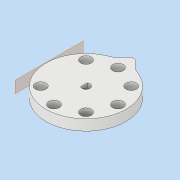
# Autodesk Inventor part: servo horn
Saved by Autodesk Inventor 2017 SP1 (Build 210196100, 196)
## iProperties
Created: 2018-12-30
Part Number: servo horn
Material: Generic
Document SubType Name: Modeling
Designer: Dylan Rice
Density: 1 g/cm^3
Appearance: Default
Author: Dylan Rice
Autodesk Inventor part; units mm, degrees
ref_plane "XZ Plane" through (0, 0, 0) normal (0, 1, 0) x (-1, 0, 0)
ref_plane "XY Plane" through (0, 0, 0) normal (0, 0, 1) x (1, 0, 0)
sketch "Sketch1" plane through (0, 0, 0) normal (0, 1, 0) x (-1, 0, 0)
  arc A0 (0.8292, 1.25) -> (0.8292, -1.25) centre (0, 0) ccw
  line L0 (0.8292, 1.25) -> (0.8292, -1.25)
  circle A1 centre (0, 0) radius 15 construction
  circle A2 centre (0, 0) radius 18 construction
  line L1 (0, -15) -> (0, -18) construction
  arc A3 (-1, -17.618) -> (1, -17.618) centre (0, -16.5) ccw
  spline S0 degree 3 poles (1, -17.618) (2.3167, -16.4404) (3.2766, -14.7515) (5, -14.1421) knots 0 0 0 0 1 1 1 1
  spline S1 degree 3 poles (-1, -17.618) (-2.3167, -16.4404) (-3.2766, -14.7515) (-5, -14.1421) knots 0 0 0 0 1 1 1 1
  arc A4 (5, -14.1421) -> (-5, -14.1421) centre (0, 0) ccw
  line L2 (0, 0) -> (13.7006, 0) construction
  line L3 (0, 0) -> (0, -3.6917) construction
  circle A5 centre (-12, 0) radius 2
  circle A6 centre (-8.4853, -8.4853) radius 2
  circle A7 centre (0, -12) radius 2
  circle A8 centre (8.4853, -8.4853) radius 2
  circle A9 centre (12, 0) radius 2 construction
  circle A10 centre (8.4853, 8.4853) radius 2
  circle A11 centre (0, 12) radius 2
  circle A12 centre (-8.4853, 8.4853) radius 2
  dimension "d50" = 36
  dimension "d0" = 3
  dimension "d1" = 2.5
  dimension "d2" = 30
  dimension "d7" = 5
  dimension "d8" = 1
  dimension "d9" = 5
  dimension "d29" = 12
  dimension "d30" = 4
  dimension "d33" = 360
  constraints: 12 centre point, 10 point on circle, 8 end point, 4 coincident, 3 vertical, 2 point on line, 1 horizontal, 1 midpoint, 1 symmetric about line, 1 vertical alignment, 28 other
  measures "d0" diameter of A0
  measures "d1" distance of L0.start L0.end
  measures "d2" diameter of A1
  measures "d7" horizontal distance of A1.end A3.centre
  measures "d8" horizontal distance of A3.end A3.centre
  measures "d9" distance from line of L1 A4.end
  measures "d29" distance of A5.centre point (0, 0)
  measures "d30" diameter of A5
extrude "Extrusion1" add sketch "Sketch1" along normal blind 4
ref_plane "Work Plane1" through (-15, 0, 0) normal (1, 0, 0) x (0, 1, 0)
ref_plane "Work Plane2" through (-15, 0, 0) normal (1, 0, 0) x (0, 1, 0)
sketch "Sketch6" plane through (-15, 0, 0) normal (1, 0, 0) x (0, 1, 0)
  line L0 (4, -14.1421) -> (4, 15) construction
  line L1 (0, 15) -> (0, -14.1421) construction
  line L2 (0, 0) -> (4, 0) construction
  circle A0 centre (2, 0) radius 1.75
  dimension "d41" = 3.5
  constraints: 2 end point, 1 centre point, 1 midpoint, 1 perpendicular, 1 point on line
  measures "d41" diameter of A0
extrude "Extrusion6" cut sketch "Sketch6" along normal blind 1.2
sketch "Sketch8" plane through (-15, 0, 0) normal (1, 0, 0) x (0, 1, 0)
  circle A0 centre (2, 0) radius 0.8
  point P0 (0, 0)
  dimension "d47" = 1.6
  constraints: 1 centre point, 1 coincident
  measures "d47" diameter of A0
extrude "Extrusion8" cut sketch "Sketch8" along normal up to surface (14.1708 mm away)
body "Solid1"
